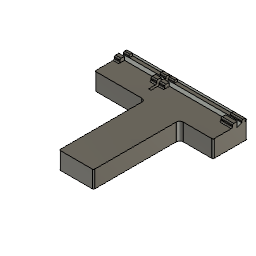
PL Hypodermic Needle Cutting Jig (Autodesk Fusion 360 design; units mm, degrees)
Autodesk Fusion 360 part; units mm, degrees
note: some values were not read from the file. Set by a fixed rule: which sketch regions a step uses; the direction of a hole.
sketch "Sketch1" plane through (0, 0, 0) normal (0, 0, 1) x (1, 0, 0) in component "Base Plate"
  line L0 (30, 25) -> (-30, 25)
  line L1 (-30, 25) -> (-30, -25)
  line L2 (-30, -25) -> (30, -25)
  line L3 (30, -25) -> (30, 25)
  line L4 (30, 25) -> (-30, -25) construction
  line L5 (-30, 25) -> (30, -25) construction
  line L6 (15, 25) -> (-15, 25) construction
  line L7 (-15, 25) -> (-15, -25) construction
  line L8 (-15, -25) -> (15, -25) construction
  line L9 (15, -25) -> (15, 25) construction
  line L10 (15, 25) -> (-15, -25) construction
  line L11 (-15, 25) -> (15, -25) construction
  line L12 (7.5, 12.5) -> (-7.5, 12.5) construction
  line L13 (-7.5, 12.5) -> (-7.5, -12.5) construction
  line L14 (-7.5, -12.5) -> (7.5, -12.5) construction
  line L15 (7.5, -12.5) -> (7.5, 12.5) construction
  line L16 (7.5, 12.5) -> (-7.5, -12.5) construction
  line L17 (-7.5, 12.5) -> (7.5, -12.5) construction
  circle A0 centre (7.5, 12.5) radius 2.25
  circle A1 centre (7.5, -12.5) radius 2.25
  circle A2 centre (-7.5, -12.5) radius 2.25
  circle A3 centre (-7.5, 12.5) radius 2.25
  circle A4 centre (-22.5, 12.7) radius 3.25
  line L18 (-15, 0) -> (-30, 0) construction
  line L19 (-22.5, 0) -> (-22.5, 12.7) construction
  line L20 (0, 0) -> (0, 25) construction
  circle A5 centre (-22.5, -12.7) radius 3.25
  circle A6 centre (22.5, 12.7) radius 3.25
  circle A7 centre (22.5, -12.7) radius 3.25
  dimension "d1" = 60
  dimension "d2" = 50
  dimension "d3" = 30
  dimension "d4" = 15
  dimension "d5" = 25
  dimension "d6" = 4.5
  dimension "d8" = 12.7
  dimension "d9" = 6.5
  constraint horizontal L0
  constraint perpendicular L0 L1
  constraint parallel L0 L2
  constraint parallel L1 L3
  constraint coincident L4 L20.start
  constraint coincident L5 L20.start
  constraint coincident L20.start origin
  constraint horizontal L6
  constraint perpendicular L6 L7
  constraint parallel L6 L8
  constraint parallel L7 L9
  constraint coincident L10 L20.start
  constraint coincident L11 L20.start
  constraint coincident L0 L6.start
  constraint horizontal L12
  constraint perpendicular L12 L13
  constraint parallel L12 L14
  constraint parallel L13 L15
  constraint coincident L16 L20.start
  constraint coincident L17 L20.start
  constraint coincident L12.start L15.end
  constraint coincident L14.end L15.start
  constraint coincident L13.end L14.start
  constraint coincident L12.end L13.start
  constraint equal A0 A3
  constraint equal A0 A1
  constraint equal A1 A2
  constraint midpoint L7 L18.start
  constraint midpoint L1 L18.end
  constraint midpoint L18 L19.start
  constraint perpendicular L18 L19
  constraint coincident A4.centre L19.end
  constraint midpoint L6 L20.end
  constraint symmetric A4 L18 A5
  constraint symmetric A4 L20 A6
  constraint symmetric L20 A5 A7
  measures "d1" distance of L0.start L0.end
  measures "d2" distance of L0.start L2.end
  measures "d3" distance of L7 L9
  measures "d4" distance of L13.end L14.end
  measures "d5" distance of L12.end L13.end
  measures "d6" diameter of A0
  measures "d8" distance of L19.start A4.centre
  measures "d9" diameter of A4
extrude "Extrude1" add sketch "Sketch1" along normal blind 8.5 makes body 1 in component "Base Plate"
sketch "Sketch2" plane through (0, 0, 0) normal (0, 0, -1) x (1, 0, 0) in component "Base Plate"
  circle A0 centre (7.5, -12.5) radius 2.25
  circle A1 centre (7.5, 12.5) radius 2.25
  circle A2 centre (-7.5, 12.5) radius 2.25
  circle A3 centre (22.5, -12.7) radius 3.25
  circle A4 centre (22.5, 12.7) radius 3.25
  circle A5 centre (-22.5, 12.7) radius 3.25
  circle A6 centre (-7.5, -12.5) radius 2.25
  circle A7 centre (-22.5, -12.7) radius 3.25
  line L0 (30, -25) -> (30, 25)
  line L1 (30, 25) -> (-30, 25)
  line L2 (-30, 25) -> (-30, -25)
  line L3 (-30, -25) -> (30, -25)
  circle A8 centre (7.5, -12.5) radius 3.75
  circle A9 centre (-7.5, -12.5) radius 3.75
  circle A10 centre (-7.5, 12.5) radius 3.75
  circle A11 centre (7.5, 12.5) radius 3.75
  dimension "d12" = 7.5
  constraint concentric A0 A8
  constraint concentric A6 A9
  constraint concentric A2 A10
  constraint concentric A1 A11
  constraint equal A10 A11
  constraint equal A8 A10
  constraint equal A8 A9
  measures "d12" diameter of A8
extrude "Extrude2" cut sketch "Sketch2" against normal blind 4.25 contours A8 | A9 | A10 | A11 bodies 1 in component "Base Plate"
fillet "Fillet1" radius 1 4 edges at (30, -25, 4.25) (30, 25, 4.25) (-30, 25, 4.25) (-30, -25, 4.25) on bodies 1 in component "Base Plate"
sketch "Sketch1 (2)" plane through (0, 0, 0) normal (0, 0, 1) x (1, 0, 0) in component "Table"
  line L0 (10, 25) -> (-10, 25) construction
  line L1 (-10, 25) -> (-10, -25) construction
  line L2 (-10, -25) -> (10, -25) construction
  line L3 (10, -25) -> (10, 25) construction
  line L4 (10, 25) -> (-10, -25) construction
  line L5 (-10, 25) -> (10, -25) construction
  line L6 (15, 40) -> (-15, 40) construction
  line L7 (-15, 40) -> (-15, -40) construction
  line L8 (-15, -40) -> (15, -40) construction
  line L9 (15, -40) -> (15, 40) construction
  line L10 (15, 40) -> (-15, -40) construction
  line L11 (-15, 40) -> (15, -40) construction
  line L12 (-59, 65) -> (-59, 35)
  line L13 (-15, -40) -> (15, -40)
  line L14 (44, 35) -> (44, 65)
  line L15 (-22, 65) -> (-20, 65)
  line L16 (-20, 65) -> (-20, 45)
  line L17 (-20, 45) -> (-22, 45)
  line L18 (-22, 45) -> (-22, 65)
  line L19 (-15, -40) -> (-15, 35)
  line L20 (15, -40) -> (15, 35)
  line L21 (15, 35) -> (44, 35)
  line L22 (-15, 35) -> (-59, 35)
  line L23 (44, 65) -> (-59, 65)
  point P0 (-10, 25)
  point P1 (10, 25)
  point P2 (10, -25)
  point P3 (-10, -25)
  dimension "d18" = 20
  dimension "d19" = 50
  dimension "d20" = 30
  dimension "d21" = 80
  dimension "d25" = 5
  dimension "d26" = 2
  dimension "d27" = 20
  dimension "d74" = 37
  dimension "d76" = 64
  dimension "d77" = 10
  dimension "d105" = 5
  constraint horizontal L0
  constraint perpendicular L0 L1
  constraint parallel L0 L2
  constraint parallel L1 L3
  constraint coincident L4 origin
  constraint coincident L5 origin
  constraint coincident P0 L0.end
  constraint coincident L0.start L3.end
  constraint coincident P2 L2.end
  constraint coincident L1.end L2.start
  constraint horizontal L6
  constraint perpendicular L6 L7
  constraint parallel L6 L8
  constraint parallel L7 L9
  constraint coincident L10 origin
  constraint coincident L11 origin
  constraint parallel L12 L14
  constraint horizontal L15
  constraint vertical L16
  constraint horizontal L17
  constraint vertical L18
  constraint vertical L19
  constraint vertical L20
  constraint horizontal L21
  constraint equal L19 L20
  constraint collinear L7 L19
  constraint coincident L8.end L9.start
  constraint coincident L7.end L8.start
  constraint perpendicular L12 L22
  constraint equal L12 L14
  constraint collinear L15 L23
  measures "d18" distance of L1.end P2
  measures "d19" distance of P0 L1.end
  measures "d20" distance of L7.end L8.end
  measures "d21" distance of L6.end L7.end
  measures "d25" distance of L7 L16
  measures "d26" distance of L16 L18
  measures "d27" distance of L15.start L17.end
  measures "d74" distance of L12 L18
  measures "d76" distance of L14 L16
  measures "d77" distance of L17 L22
  measures "d105" distance of L6 L21
extrude "Extrude1'" add sketch "Sketch1 (2)" along normal blind 15 separate body contours L12 L13 L14 L16 L17 L18 L19 L20 L21 L22 L23 makes body 2 in component "Table"
sketch "Sketch2 (2)" plane through (44, 0, 0) normal (1, 0, 0) x (0, 1, 0) in component "Table"
  line L0 (35, 0) -> (65, 0)
  line L1 (65, 15) -> (35, 15)
  line L2 (35, 15) -> (35, 0)
  line L3 (65, 15) -> (63, 14.2929)
  line L4 (63, 14.2929) -> (63, 15)
  circle A0 centre (63.5, 15) radius 0.5 construction
  line L5 (63, 15) -> (60, 15)
  line L6 (60, 15) -> (60, 17)
  line L7 (60, 17) -> (63, 17)
  line L8 (63, 17) -> (63, 15)
  line L9 (56, 15) -> (52, 15)
  line L10 (56, 18) -> (56, 15)
  line L11 (52, 18) -> (56, 18)
  line L12 (52, 15) -> (52, 18)
  circle A1 centre (57.125, 15) radius 1.125 construction
  line L13 (60, 15) -> (56, 13.2992)
  line L14 (56, 13.2992) -> (56, 15)
  line L15 (65, 0) -> (65, 15)
  line L16 (65, 5) -> (52, 5) construction
  dimension "d52" = 1
  dimension "d78" = 2
  dimension "d81" = 2.25
  dimension "d82" = 3
  dimension "d83" = 4
  dimension "d84" = 4
  dimension "d85" = 3
  dimension "d106" = 13
  dimension "d108" = 10
  constraint vertical L4
  constraint tangent L3 A0
  constraint horizontal L5
  constraint vertical L6
  constraint horizontal L7
  constraint vertical L8
  constraint collinear L1 L5
  constraint tangent L4 A0
  constraint vertical L14
  constraint tangent A1 L13
  constraint horizontal L9
  constraint vertical L12
  constraint horizontal L11
  constraint vertical L10
  constraint tangent A1 L14
  constraint collinear L1 L9
  constraint coincident L15 L16.start
  constraint perpendicular L15 L16
  constraint vertical L11.start L16.end
  constraint coincident L1 A1.centre
  constraint coincident L1 A0.centre
  constraint coincident L1.start L3.start
  measures "d52" diameter of A0
  measures "d78" distance of L4.end L7.end
  measures "d81" diameter of A1
  measures "d82" distance of L9.start L10.start
  measures "d83" distance of L11.start L10.start
  measures "d84" distance of L6 L10
  measures "d85" distance of L6.end L7.end
  measures "d106" distance of L16.start L16.end
  measures "d108" distance of L1 L16
hole "Hole1" at (10, -25, 0) at (-10, -25, 0) at (-10, 25, 0) at (10, 25, 0) direction (0, 0, 1) diameter 4.527 depth 6.03 tip angle 90 countersink diameter 5.23 countersink angle 50 bodies 2 in component "Table"
extrude "Extrude8" cut sketch "Sketch2 (2)" against normal blind 103 contours L1 L3 L4 | L1 L13 L14 bodies 2 in component "Table"
extrude "Extrude9" add sketch "Sketch2 (2)" against normal blind 10 contours L1 L9 L10 L11 L12 | L1 L5 L6 L7 L8 bodies 2 in component "Table"
extrude "Extrude10" add sketch "Sketch2 (2)" along normal blind 5 from surface at -64 contours L1 L9 L10 L11 L12 | L1 L5 L6 L7 L8 bodies 2 in component "Table"
extrude "Extrude11" add sketch "Sketch2 (2)" against normal blind 5 from surface at -66 contours L1 L9 L10 L11 L12 | L1 L5 L6 L7 L8 bodies 2 in component "Table"
extrude "Extrude12" add sketch "Sketch2 (2)" along normal blind 5 from surface at -103 contours L1 L9 L10 L11 L12 | L1 L5 L6 L7 L8 bodies 2 in component "Table"
fillet "Fillet4" radius 1 12 edges at (39, 52, 15) (39, 52, 18) (-17.5, 52, 15) (-17.5, 52, 18) (-24.5, 52, 15) (-24.5, 52, 18) (-56.5, 52, 15) (-56.5, 52, 18) (-17.5, 60, 17) (-24.5, 60, 17) (-56.5, 60, 17) (39, 60, 17) on bodies 2 in component "Table"
fillet "Fillet5" radius 1 6 edges at (-59, 35, 7.5) (-15, -40, 7.5) (15, -40, 7.5) (44, 35, 7.5) (44, 65, 7.5) (-59, 65, 7.5) on bodies 2 in component "Table"
fillet "Fillet6" radius 3 2 edges at (15, 35, 7.5) (-15, 35, 7.5) on bodies 2 in component "Table"
component "Base Plate" placed x (1, 0, 0) y (0, 1, 0) z (0, 0, 1) at (0, 0, 0)
component "Table" placed x (1, 0, 0) y (0, 1, 0) z (0, 0, 1) at (0, 0, 0)
equation "d8 = 1 in / 2"
equation "d69 = 5.03 mm + 1 mm"
equation "d70 = ( 5.03 * 0.9 ) * 1 mm"
equation "d72 = 5.03 mm + 0.2 mm"
equation "d74 = 27 mm + ( ( 2 * 5 ) * 1 mm )"
equation "d76 = ( ( 27 * 2 ) * 1 mm ) + ( ( 2 * 5 ) * 1 mm )"
